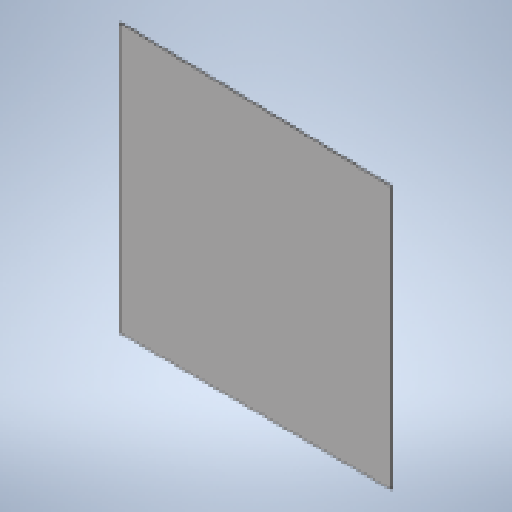
# Autodesk Inventor part: GBK 2331 shield 9
Saved by Autodesk Inventor 2026 (Build 300175000, 175)
## iProperties
Created: 2026-04-17
Part Number: GBK 2331 shield 9
Material: Steel
Document SubType Name: Sheet Metal
Designer: pokla
Stock Number: 2339
Mass: 69243.3 g
Surface Area: 44341.6 cm^2
Volume: 8820.8 cm^3
Density: 7.85 g/cm^3
Flat Pattern Width: 148 cm
Flat Pattern Length: 146.5 cm
Flat Pattern Area: 21682 cm^2
Sheet Metal Rule: По умолчанию_мм
Sheet Metal Width: 1480,000 мм
Sheet Metal Length: 1465,000 мм
Sheet Metal Area: 2168200,000 мм^2
Appearance: Default
Author: admin
Autodesk Inventor part; units mm, degrees
ref_plane "YZ Plane" through (0, 0, 0) normal (1, 0, 0) x (0, 1, 0)
ref_plane "XZ Plane" through (0, 0, 0) normal (0, 1, 0) x (-1, 0, 0)
ref_plane "XY Plane" through (0, 0, 0) normal (0, 0, 1) x (1, 0, 0)
sketch "Sketch1" plane through (0, 0, 0) normal (0, 0, 1) x (1, 0, 0)
  line L0 (740, -745) -> (-740, -745)
  line L1 (-740, -745) -> (-740, 745)
  line L2 (-740, 745) -> (740, 745)
  line L3 (740, 745) -> (740, -745)
  line L4 (740, -745) -> (-740, 745) construction
  line L5 (-740, -745) -> (740, 745) construction
  line L6 (-740, 720) -> (740, 686.4141)
  point P0 (0, 0)
  dimension "d0" = 1480
  dimension "d1" = 1490
  dimension "d3" = 1.3
  dimension "d8" = 1465
  measures "d0" distance of L1.end L2.end
  measures "d1" distance of L0.end L1.end
  measures "d3" angle of L2 L6
  measures "d8" distance of L6.start L0.end
extrude "Plate1" add sketch "Sketch1" along normal blind 4 contours L0 L1 L6 L3
sketch "Эскиз2" plane through (0, 0, 0) normal (0, 0, -1) x (-1, 0, 0)
  line L0 (566.7109, -523.3382) -> (566.7109, -1021.4744) construction
  line L1 (566.7109, -1021.4744) -> (527.0836, -1021.4744) construction
  line L2 (527.0836, -1021.4744) -> (527.0836, -523.3382) construction
  line L3 (527.0836, -523.3382) -> (566.7109, -523.3382) construction
  line L4 (710, -489.5) -> (710, -485.5) projected
  line L5 (710, 7.1667) -> (710, 11.1667) projected
  line L6 (710, 503.8333) -> (710, 507.8333) projected
  line L7 (210.5058, -493) -> (210.5058, -590) projected
  line L8 (210.5058, -590) -> (206.5068, -590) projected
  line L9 (-289.6228, -493) -> (-289.6228, -590) projected
  line L10 (-289.6228, -590) -> (-293.6218, -590) projected
  line L11 (-739.3197, -489.5) -> (-710, -489.5) projected
  line L12 (-710, -489.5) -> (-710, -485.5) projected
  line L13 (-739.3197, 7.1667) -> (-710, 7.1667) projected
  line L14 (-710, 7.1667) -> (-710, 11.1667) projected
  line L15 (-739.3197, 503.8333) -> (-710, 503.8333) projected
  line L16 (-710, 503.8333) -> (-710, 507.8333) projected
  line L17 (-289.6228, 715) -> (-289.6228, 511) projected
  line L18 (210.5058, 715) -> (210.5058, 511) projected
  line L19 (710, -489.5) -> (680, -489.5)
  line L20 (710, 7.1667) -> (680, 7.1667)
  line L21 (710, 503.8333) -> (680, 503.8333)
  point P0 (0, 0)
  dimension "d5" = 30
  dimension "d9" = 30
  dimension "d10" = 30
  constraints: 6 end point, 3 horizontal, 2 other
  measures "d5" distance of L4.start L19.end
  measures "d9" distance of L5.start L20.end
  measures "d10" distance of L6.start L21.end
mark "Маркировка1"
equation "\"d0\" = Лист_ширина"
equation "\"d2\" = Thickness"
equation "\"BendRadius\" = Thickness"
equation "\"BendReliefWidth\" = Thickness"
equation "\"BendReliefDepth\" = 0.5 * Thickness"
equation "\"CornerReliefSize\" = 4 * Thickness"
equation "\"MinimumRemnant\" = 2 * Thickness"
equation "\"TransitionRadius\" = BendRadius"
equation "\"JacobiRadiusSize\" = BendRadius"
equation "\"GapSize\" = Thickness"
equation "\"Лист_ширина\" = 1480"
equation "\"Thickness\" = 4"
body "Solid1"
